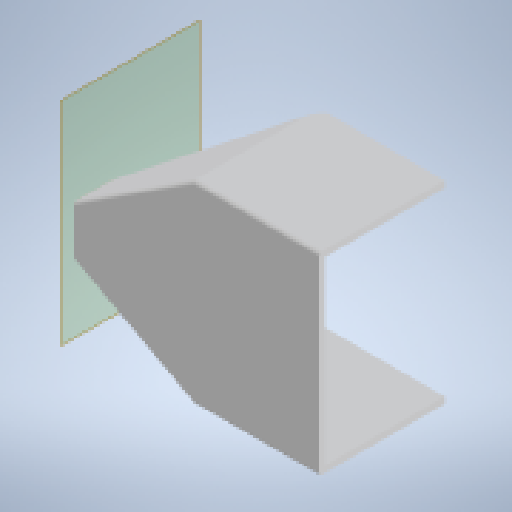
# Autodesk Inventor part: WingBoxCouple
Saved by Autodesk Inventor 2026 (Build 300175050, 175E)
## iProperties
Created: 2025-07-20
Part Number: WingBoxCouple
Material: Generic
Document SubType Name: Modeling
Designer: Cupri
Density: 1 g/cm^3
Appearance: Default
Author: Cupri
Autodesk Inventor part; units mm, degrees
ref_plane "YZ Plane" through (0, 0, 0) normal (1, 0, 0) x (0, 1, 0)
ref_plane "XZ Plane" through (0, 0, 0) normal (0, 1, 0) x (-1, 0, 0)
ref_plane "XY Plane" through (0, 0, 0) normal (0, 0, 1) x (1, 0, 0)
sketch "Sketch14" plane through (0, 0, 0) normal (1, 0, 0) x (0, 1, 0)
  line L0 (0, 4.9685) -> (-195, 4.9685)
  line L1 (-195, 4.9685) -> (-195, -122.0315)
  line L2 (-195, -122.0315) -> (0, -122.0315)
  line L3 (0, -122.0315) -> (0, 4.9685)
  line L4 (-6.35, -1.3815) -> (-188.65, -1.3815)
  line L5 (-188.65, -1.3815) -> (-188.65, -115.6815)
  line L6 (-188.65, -115.6815) -> (-6.35, -115.6815)
  line L7 (-6.35, -115.6815) -> (-6.35, -1.3815)
  line L8 (0, 4.9685) -> (-195, 4.9685)
  point P0 (0, 0)
  constraints: 18 end point
extrude "Extrusion10" add sketch "Sketch14" against normal blind 127
ref_plane "Work Plane11" through (-254, 0, 0) normal (-1, 0, 0) x (0, 0, 1)
sketch "Sketch19" plane through (-254, 0, 0) normal (-1, 0, 0) x (0, 0, 1)
  line L0 (-52.1815, -135.6) -> (-1.3815, -135.6)
  line L1 (-1.3815, -135.6) -> (-1.3815, -84.8)
  line L2 (-1.3815, -84.8) -> (-52.1815, -84.8)
  line L3 (-52.1815, -84.8) -> (-52.1815, -135.6)
  line L4 (-115.6815, -110.2) -> (0, -110.2) construction
  line L5 (-1.3815, -6.35) -> (-1.3815, -188.65) projected
  point P0 (0, 0)
  point P1 (-52.1815, -110.2)
  point P2 (-45.8315, -188.65)
  point P3 (-26.7815, -135.6)
  dimension "d56" = 50.8
  dimension "d57" = 50.8
  dimension "d59" = 0
  dimension "d71" = 0
  constraints: 10 end point, 2 horizontal, 2 midpoint, 2 parallel, 1 perpendicular
  measures "d56" distance of L2.end L1.end
  measures "d57" distance of L1.end L0.end
  measures "d59" distance from line of L4 point (-52.181, -110.2)
  measures "d71" distance between parallel lines of L5 L1
loft "Loft1" add profiles "Sketch19" section 2 edges at (-127, -97.5, 4.9685) (-127, 0, -58.5315) (-127, -97.5, -122.0315) (-127, -195, -58.5315)
shell "Shell2" thickness 7.3025 removed faces 1 at (-127, -127.8833, -39.4815)
sketch "Sketch20" plane through (0, -195, -122.0315) normal (0, 0, -1) x (-1, 0, 0)
  line L0 (0, 0) -> (0, 195) projected
  line L1 (0, 0) -> (127, 0) projected
  line L2 (127, 195) -> (127, 0) projected
  line L3 (0, 195) -> (127, 195) projected
  line L4 (0, 6.35) -> (127, 6.35) projected
  line L5 (0, 188.65) -> (127, 188.65) projected
  line L6 (127, 188.65) -> (127, 6.35) projected
  line L7 (120.65, 6.35) -> (127, 6.35)
  line L8 (127, 6.35) -> (127, 188.65)
  line L9 (127, 188.65) -> (120.65, 188.65)
  line L10 (120.65, 188.65) -> (120.65, 6.35)
  dimension "d67" = 6.35
  constraints: 8 end point, 2 parallel, 1 horizontal, 1 perpendicular, 1 point on line
  measures "d67" distance between parallel lines of L2 L10
extrude "Extrusion15" cut sketch "Sketch20" against normal up to surface (6.35 mm away) contours L0 L5 L10 L4
fillet "Fillet3" radius 19.05 2 edges at (-190.5, -42.4, -87.1065) (-190.5, -165.3, -87.1065)
fillet "Fillet4" radius 3.175 4 edges at (-190.5, -42.4, 1.7935) (-63.5, 0, 4.9685) (-190.5, -165.3, 1.7935) (-63.5, -195, 4.9685)
body "Solid2"
